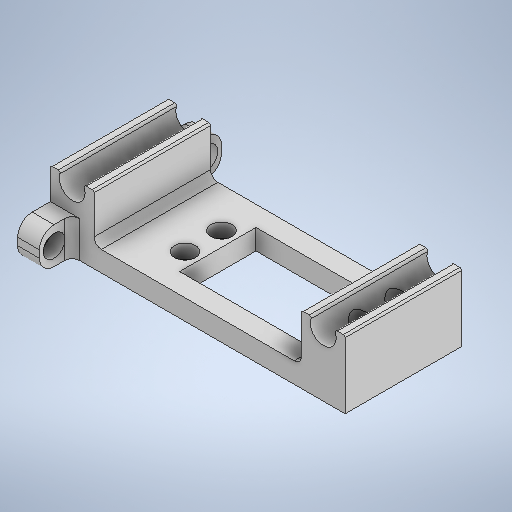
# Autodesk Inventor part: Servo mount - fron
Saved by Autodesk Inventor 2025.2 (Build 292293000, 293)
## iProperties
Created: 2025-01-30
Part Number: Servo mount - fron
Material: Generic
Document SubType Name: Modeling
Designer: caomi
Density: 1 g/cm^3
Appearance: Default
Author: caomi
Autodesk Inventor part; units mm, degrees
ref_plane "YZ Plane" through (0, 0, 0) normal (1, 0, 0) x (0, 1, 0)
ref_plane "XZ Plane" through (0, 0, 0) normal (0, 1, 0) x (-1, 0, 0)
ref_plane "XY Plane" through (0, 0, 0) normal (0, 0, 1) x (1, 0, 0)
sketch "Sketch1" plane through (0, 0, 0) normal (0, 1, 0) x (-1, 0, 0)
  line L0 (-20, -10) -> (20, -10)
  line L1 (20, -10) -> (20, 10)
  line L2 (20, 10) -> (-20, 10)
  line L3 (-20, 10) -> (-20, -10)
  line L4 (-20, -10) -> (20, 10) construction
  line L5 (20, -10) -> (-20, 10) construction
  circle A0 centre (10, 0) radius 2.6964
  circle A1 centre (24.5, 5) radius 2
  circle A2 centre (24.5, -5) radius 2
  line L6 (66.7, 0) -> (-46.7, 0) projected
  circle A3 centre (-24.5, 5) radius 2
  circle A4 centre (-24.5, -5) radius 2
  line L7 (50.5, 16) -> (-30.5, 16)
  line L8 (-30.5, 16) -> (-30.5, -16)
  line L9 (-30.5, -16) -> (50.5, -16)
  line L10 (50.5, -16) -> (50.5, 16)
  line L11 (10, 6.1182) -> (10, -6.1182) construction
  line L12 (-28.5, 14.25) -> (-28.5, 16)
  line L13 (20.5, 10.5) -> (20.5, -10.5)
  line L14 (20.5, -10.5) -> (-20.5, -10.5)
  line L15 (-20.5, -10.5) -> (-20.5, 10.5)
  line L16 (-20.5, 10.5) -> (20.5, 10.5)
  point P0 (0, 0)
  point P1 (-20.5, 0)
  point P2 (20.5, 0)
  point P3 (20, 0)
  point P4 (-20, 0)
  dimension "d0" = 40
  dimension "d1" = 20
  dimension "d2" = 30
  dimension "d3" = 10
  dimension "d4" = 4.5
  dimension "d5" = 10
  dimension "d6" = 4.5
  dimension "d7" = 4
  dimension "d8" = 6
  dimension "d9" = 6
  dimension "d31" = 0.5
  constraints: 32 end point, 6 parallel, 5 centre point, 4 perpendicular, 3 midpoint, 2 coincident, 2 horizontal, 2 point on line, 1 equal radius, 1 vertical, 7 other
  measures "d0" distance of L1.end L2.end
  measures "d1" distance of L0.end L1.end
  measures "d2" distance from line of L3 A0.centre
  measures "d3" distance of A1.centre A2.centre
  measures "d4" distance from line of L1 A1.centre
  measures "d5" distance of A3.centre A4.centre
  measures "d6" distance from line of L3 A3.centre
  measures "d7" diameter of A1
  measures "d8" distance from line of A3.centre L8
  measures "d9" distance between parallel lines of L9 L0
  measures "d31" distance between parallel lines of L1 L13
extrude "Base" add sketch "Sketch1" along normal blind 5.6 contours L15 L14 L13 L6 L10 L9 L8 | L6 L8 L7 L10 L13 L16 L15 | A1 | A2 | A3 | A4
sketch "Sketch3" plane through (0, 5.6, 0) normal (0, 1, 0) x (1, 0, 0)
  line L0 (-66.7, 0) -> (46.7, 0) projected
  line L1 (0, -6.8326) -> (0, 7.3627) construction
  circle A0 centre (24.5, -5) radius 2.9
  circle A1 centre (24.5, 5) radius 2.9
  circle A2 centre (-24.5, -5) radius 2.9
  circle A3 centre (-24.5, 5) radius 2.9
  line L2 (20, -10) -> (20, 10) projected
  point P0 (0, 0)
  dimension "d19" = 10
  dimension "d28" = 5.8
  dimension "d32" = 4.5
  constraints: 4 centre point, 4 coincident, 3 equal radius, 3 symmetric about line, 2 end point, 1 point on line, 1 vertical, 1 vertical alignment
  measures "d19" distance of point (24.5, 5) point (24.5, -5)
  measures "d28" diameter of A0
  measures "d32" distance from line of A0.centre L2
hole "Servo mount holes" at (24.5, 5.6, 5) at (24.5, 5.6, -5) at (-24.5, 5.6, 5) at (-24.5, 5.6, -5) direction (0, -1, 0) diameter 4.3 end through all counterbore diameter 5.8 counterbore depth 4
sketch "Sketch2" plane through (-50.5, 0, 16) normal (0, 0, 1) x (1, 0, 0)
  line L0 (81, 5.6) -> (0, 5.6) projected
  line L1 (0, 5.6) -> (12, 5.6)
  line L2 (12, 5.6) -> (12, 18.6)
  line L3 (12, 18.6) -> (0, 18.6)
  line L4 (0, 18.6) -> (0, 5.6)
  circle A0 centre (6, 16.8) radius 3.55
  circle A1 centre (6, 16.8) radius 3.05
  line L5 (40.5, 13.1003) -> (40.5, -16.3877) construction
  line L6 (81, 5.6) -> (69, 5.6)
  line L7 (69, 5.6) -> (69, 18.6)
  line L8 (69, 18.6) -> (81, 18.6)
  line L9 (81, 18.6) -> (81, 5.6)
  circle A2 centre (75, 16.8) radius 3.55
  circle A3 centre (75, 16.8) radius 3.05
  line L10 (2.45, 16.8) -> (9.55, 16.8)
  line L11 (78.55, 16.8) -> (71.45, 16.8)
  point P0 (50.5, 0)
  point P1 (9.0598, 18.6)
  point P2 (2.9402, 18.6)
  point P3 (8.4622, 18.6)
  point P4 (3.5378, 18.6)
  point P5 (6, 18.6)
  point P6 (40.5, 5.6)
  point P7 (75, 18.6)
  point P8 (78.0598, 18.6)
  point P9 (71.9402, 18.6)
  point P10 (72.5378, 18.6)
  point P11 (77.4622, 18.6)
  point P12 (71.95, 16.8)
  point P13 (78.05, 16.8)
  point P14 (9.05, 16.8)
  point P15 (2.95, 16.8)
  dimension "d12" = 12
  dimension "d13" = 13
  dimension "d14" = 7.1
  dimension "d33" = 0.5
  dimension "d38" = 1.8
  constraints: 22 end point, 8 symmetric about line, 4 centre point, 3 coincident, 3 midpoint, 2 horizontal, 2 parallel, 2 point on circle, 1 perpendicular, 1 point on line, 1 vertical, 1 vertical alignment, 2 other
  measures "d12" distance of L2.end L3.end
  measures "d13" distance between parallel lines of L0 L3
  measures "d14" diameter of A0
  measures "d33" radial gap between concentric circles of A0 A1
  measures "d38" distance from line of L3 A0.centre
extrude "Linear rod mount" add sketch "Sketch2" against normal up to surface (32 mm away) contours L0 L4 L3 A0 L2 | L0 L7 L8 A2 L9
extrude "Servo mount hole extended" cut sketch "Sketch3" along normal blind 10 contours A0 | A1
fillet "Fillet1" radius 2 3 edges at (-38.5, 5.6, 0) (18.5, 5.6, 13.25) (18.5, 5.6, -13.25)
fillet "Fillet2" radius 0.5 8 edges at (-50.5, 18.6, 0) (-38.5, 18.6, 0) (18.5, 18.6, 0) (30.5, 18.6, 0) (-47.5598, 18.6, 0) (-41.4402, 18.6, 0) (21.4402, 18.6, 0) (27.5598, 18.6, 0)
sketch "Sketch4" plane through (0, 0, 0) normal (0, 0, 1) x (1, 0, 0)
  line L0 (-50.5, 0) -> (-44.5, 0)
  line L1 (-44.5, 0) -> (-44.5, 10)
  line L2 (-44.5, 10) -> (-50.5, 10)
  line L3 (-50.5, 10) -> (-50.5, 0)
  point P0 (0, 0)
  dimension "d39" = 10
  dimension "d40" = 6
  constraints: 8 end point, 2 parallel, 1 horizontal, 1 perpendicular
  measures "d39" distance of L2.end L0.start
  measures "d40" distance of L0.start L0.end
extrude "Extrusion5" add sketch "Sketch4" along normal mid plane 50
fillet "Fillet3" radius 4 4 edges at (-47.5, 10, 25) (-47.5, 0, 25) (-47.5, 10, -25) (-47.5, 0, -25)
sketch "Sketch5" plane through (-44.5, 0, 16) normal (1, 0, 0) x (0, 0, -1)
  arc A0 (-5, 10) -> (-9, 6) centre (-5, 6) ccw projected
  arc A1 (41, 6) -> (37, 10) centre (37, 6) ccw projected
  line L0 (-9, 4) -> (-9, 6) projected
  line L1 (41, 6) -> (41, 4) projected
  point P0 (16, 0)
  point P1 (-5, 5)
  point P2 (37, 5)
  point P3 (-5, 0)
  point P4 (-9, 5)
  point P5 (41, 5)
  constraints: 2 horizontal alignment, 2 midpoint, 2 vertical alignment
hole "Hole2" at (-44.5, 5, 21) at (-44.5, 5, -21) direction (-1, 0, 0) diameter 4.5 end through all counterbore diameter 6 counterbore depth 4
fillet "Fillet4" radius 2 2 edges at (-44.5, 5, 16) (-44.5, 5, -16)
equation "\"d9\" = d8"
body "Solid1"
